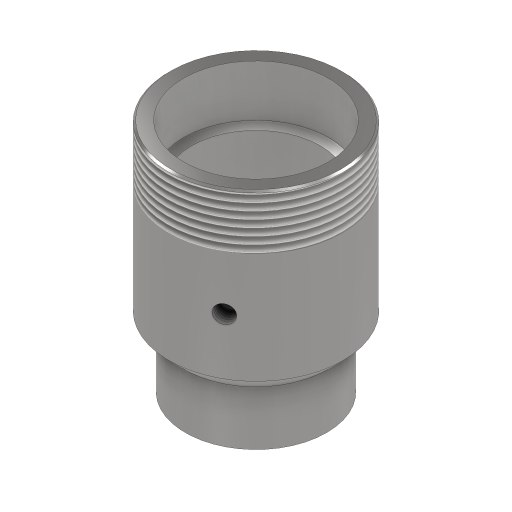
# Autodesk Inventor part: OringNut
Saved by Autodesk Inventor 2024.2 (Build 282272000, 272)
## iProperties
Created: 2022-12-02
Part Number: OringNut
Material: Stainless Steel, 440C
Document SubType Name: Modeling
Designer: kuzmin
Density: 7.75 g/cm^3
Appearance: Semi-Polished
Author: kuzmin
Autodesk Inventor part; units mm, degrees
ref_plane "XZ Plane" through (0, 0, 0) normal (0, 1, 0) x (-1, 0, 0)
ref_plane "XY Plane" through (0, 0, 0) normal (0, 0, 1) x (1, 0, 0)
sketch "Sketch3" plane through (0, 0, 0) normal (0, 0, 1) x (1, 0, 0)
  line L0 (0, 0) -> (0, 23.925) construction
  line L1 (17.75, 0) -> (17.75, 50)
  line L2 (17.75, 0) -> (19.5, 0)
  line L3 (19.5, 0) -> (19.5, 15)
  line L4 (19.5, 15) -> (24, 15)
  line L5 (24, 15) -> (24, 65)
  line L6 (17.75, 50) -> (20, 50.8189)
  line L7 (20, 50.8189) -> (20, 65)
  line L8 (20, 65) -> (24, 65)
  dimension "d9" = 35.5
  dimension "d10" = 39
  dimension "d11" = 40
  dimension "d13" = 70
  dimension "d14" = 48
  dimension "d15" = 15
  dimension "d16" = 50
  dimension "d27" = 65
  constraints: 18 end point, 3 vertical, 2 horizontal, 1 horizontal alignment, 1 perpendicular
  measures "d9" diameter of L1 L0
  measures "d10" diameter of L3 L0
  measures "d11" diameter of L7 L0
  measures "d13" angle of L1 L6
  measures "d14" diameter of L5 L0
  measures "d15" distance from line of L8 L1.end
  measures "d16" distance of L4.end L5.end
  measures "d27" distance between parallel lines of L2 L8
revolve "Revolution2" add sketch "Sketch3" angle 360 about axis through (0, 0, 0) along (0, 1, 0)
chamfer "Chamfer1" distance 4.5 angle 45 1 edges at (-24, 15, 0)
thread "Thread1" size "M48x2" class "6g" standard "ANSI Metric M Profile" length 15
chamfer "Chamfer2" distance 0.5 angle 45 1 edges at (-24, 65, 0)
ref_plane "Work Plane1" through (-24, 40, 0) normal (1, 0, 0) x (0, 1, 0)
sketch "Sketch4" plane through (-24, 40, 0) normal (1, 0, 0) x (0, 1, 0)
  circle A0 centre (-5, 0) radius 2.5
  line L0 (25, 23.5) -> (25, -23.5) projected
  point P0 (-40, 0)
  dimension "d28" = 5
  dimension "d29" = 30
  constraints: 1 centre point, 1 horizontal alignment
  measures "d28" diameter of A0
  measures "d29" distance from line of L0 A0.centre
extrude "Extrusion1" cut sketch "Sketch4" along normal blind 5
thread "Thread2" size "M5x0.8" class "6H" standard "ANSI Metric M Profile" full length
pattern_circular "Circular Pattern1" count 3 over 360 about axis through (0, 40, 0) along (0, 1, 0) of "Extrusion1"
body "Solid2"
